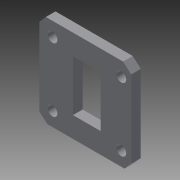
# Autodesk Inventor part: WG17FLANGE
Saved by Autodesk Inventor 2014 (Build 180170000, 170)
## iProperties
Created: 2014-03-25
Part Number: WG17FLANGE
Material: Generic
Document SubType Name: Modeling
Designer: jad211
Density: 1 g/cm^3
Appearance: Default
Author: jad211
Autodesk Inventor part; units mm, degrees
ref_plane "YZ Plane" through (0, 0, 0) normal (1, 0, 0) x (0, 1, 0)
ref_plane "XZ Plane" through (0, 0, 0) normal (0, 1, 0) x (-1, 0, 0)
ref_plane "XY Plane" through (0, 0, 0) normal (0, 0, 1) x (1, 0, 0)
sketch "Sketch3" plane through (0, 0, 0) normal (0, 0, 1) x (1, 0, 0)
  line L0 (-16.4175, -19.05) -> (15.5825, -19.05)
  line L1 (18.3411, -15.8973) -> (18.3411, 16.1027)
  line L2 (14.9996, 19.05) -> (-17.0004, 19.05)
  line L3 (-19.7589, 15.8973) -> (-19.7589, -16.1027)
  line L4 (-17.0004, 19.05) -> (-19.7589, 15.8973)
  line L5 (14.9996, 19.05) -> (18.3411, 16.1027)
  line L6 (18.3411, -15.8973) -> (15.5825, -19.05)
  line L7 (-19.7589, -16.1027) -> (-16.4175, -19.05)
  line L8 (-5.7625, -10.525) -> (5.7625, -10.525)
  line L9 (5.7625, -10.525) -> (5.7625, 10.525)
  line L10 (5.7625, 10.525) -> (-5.7625, 10.525)
  line L11 (-5.7625, 10.525) -> (-5.7625, -10.525)
  circle A0 centre (-14.25, 13.21) radius 2.045
  circle A1 centre (14.25, 13.21) radius 2.045
  circle A2 centre (-14.25, -13.21) radius 2.045
  circle A3 centre (14.25, -13.21) radius 2.045
  point P0 (0, 0)
  dimension "d10" = 11.525
  dimension "d11" = 21.05
  dimension "d12" = 4.09
  dimension "d13" = 4.09
  dimension "d17" = 4.09
  dimension "d19" = 28.5
  dimension "d21" = 4.09
  dimension "d38" = 10.525
  dimension "d39" = 5.7625
  dimension "d45" = 38.1
  dimension "d46" = 38.1
  dimension "d47" = 32
  dimension "d48" = 32
  dimension "d49" = 32
  dimension "d50" = 32
  dimension "d63" = 28.5
  dimension "d67" = 19.05
  dimension "d68" = 14.25
  dimension "d69" = 14.25
  dimension "d70" = 26.42
  dimension "d72" = 13.21
  dimension "d73" = 26.42
  dimension "d75" = 13.21
  constraints: 24 end point, 7 parallel, 4 centre point, 2 horizontal, 1 perpendicular
  measures "d10" distance of L10.end L9.end
  measures "d11" distance of L9.end L8.end
  measures "d12" diameter of A0
  measures "d13" diameter of A1
  measures "d17" diameter of A2
  measures "d19" distance of A1.centre A0.centre
  measures "d21" diameter of A3
  measures "d38" distance from line of point (0, 0) L8
  measures "d39" distance from line of point (0, 0) L9
  measures "d45" distance between parallel lines of L0 L2
  measures "d46" distance between parallel lines of L1 L3
  measures "d47" distance of L2.start L2.end
  measures "d48" distance of L3.start L3.end
  measures "d49" distance of L0.start L0.end
  measures "d50" distance of L1.start L1.end
  measures "d63" distance of A3.centre A2.centre
  measures "d67" distance from line of point (0, 0) L2
  measures "d68" horizontal distance of point (0, 0) A1.centre
  measures "d69" horizontal distance of point (0, 0) A3.centre
  measures "d70" distance of A2.centre A0.centre
  measures "d72" vertical distance of A0.centre point (0, 0)
  measures "d73" distance of A3.centre A1.centre
  measures "d75" vertical distance of point (0, 0) A1.centre
extrude "Extrusion5" add sketch "Sketch3" along normal blind 4
body "Solid4"
